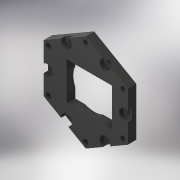
# Autodesk Inventor part: TA01
Saved by Autodesk Inventor 2017 (Build 210142000, 142)
## iProperties
Created: 2018-10-09
Part Number: TA01
Material: ABS Plastic
Document SubType Name: Modeling
Designer: Zach
Density: 1.06 g/cm^3
Appearance: Smooth - Black
Author: Zach
Autodesk Inventor part; units mm, degrees
ref_plane "YZ Plane" through (0, 0, 0) normal (1, 0, 0) x (0, 1, 0)
ref_plane "XZ Plane" through (0, 0, 0) normal (0, 1, 0) x (-1, 0, 0)
ref_plane "XY Plane" through (0, 0, 0) normal (0, 0, 1) x (1, 0, 0)
sketch "Sketch1" plane through (0, 0, 0) normal (0, 0, 1) x (1, 0, 0)
  circle A0 centre (0, 0) radius 12.5
  circle A1 centre (-30, 0) radius 3
  circle A2 centre (-15, -25.9808) radius 3
  circle A3 centre (15, -25.9808) radius 3
  circle A4 centre (30, 0) radius 3
  circle A5 centre (15, 25.9808) radius 3
  circle A6 centre (-15, 25.9808) radius 3
  line L0 (0, 57.5) -> (49.7965, 28.75)
  line L1 (49.7965, 28.75) -> (49.7965, -28.75)
  line L2 (49.7965, -28.75) -> (0, -57.5)
  line L3 (0, -57.5) -> (-49.7965, -28.75)
  line L4 (-49.7965, -28.75) -> (-49.7965, 28.75)
  line L5 (-49.7965, 28.75) -> (0, 57.5)
  point P0 (49.7965, 0)
  dimension "d0" = 25
  dimension "d2" = 6
  dimension "d6" = 360
  dimension "d15" = 30
  dimension "d33" = 115
  constraints: 12 end point, 7 centre point, 2 coincident, 2 horizontal alignment, 1 midpoint, 26 other
  measures "d0" diameter of A0
  measures "d2" diameter of A1
  measures "d15" distance of point (0, 0) A1.centre
  measures "d33" distance of L2.end L0.start
extrude "Extrusion1" add sketch "Sketch1" along normal blind 10 contours A1 | A2 | A3 | A4 | A5 | A6 | L0 L1 L2 L3 L4 L5
sketch "Sketch7" plane through (0, 0, 10) normal (0, 0, 1) x (1, 0, 0)
  circle A0 centre (0, 51) radius 3
  circle A1 centre (-44.1673, 25.5) radius 3
  circle A2 centre (-44.1673, -25.5) radius 3
  circle A3 centre (0, -51) radius 3
  circle A4 centre (44.1673, -25.5) radius 3
  circle A5 centre (44.1673, 25.5) radius 3
  line L0 (0, 51) -> (0, -51)
  point P0 (0, 0)
  dimension "d42" = 6
  dimension "d46" = 360
  dimension "d96" = 102
  constraints: 6 centre point, 2 end point, 1 vertical, 13 other
  measures "d42" diameter of A0
  measures "d96" distance of L0.start L0.end
extrude "Extrusion6" cut sketch "Sketch7" against normal through all
sketch "Sketch9" plane through (0, 0, 0) normal (0, 0, -1) x (-1, 0, 0)
  circle A0 centre (0, 0) radius 25
  dimension "d56" = 50
  constraints: 1 centre point, 1 coincident
  measures "d56" diameter of A0
extrude "Extrusion8" cut sketch "Sketch9" against normal blind 5
sketch "Sketch14" plane through (0, 0, 10) normal (0, 0, 1) x (1, 0, 0)
  circle A0 centre (-45.7965, 0) radius 2.5
  circle A1 centre (-22.8982, -39.6609) radius 2.5
  circle A2 centre (22.8982, -39.6609) radius 2.5
  circle A3 centre (45.7965, 0) radius 2.5
  circle A4 centre (22.8982, 39.6609) radius 2.5
  circle A5 centre (-22.8982, 39.6609) radius 2.5
  line L0 (-49.7965, 28.75) -> (-49.7965, -28.75) projected
  point P0 (0, 0)
  point P1 (-45.7965, 0)
  dimension "d81" = 5
  dimension "d85" = 360
  dimension "d97" = 4
  constraints: 6 centre point, 1 coincident, 1 horizontal alignment, 13 other
  measures "d81" diameter of A0
  measures "d97" distance from line of L0 A0.centre
extrude "Extrusion13" cut sketch "Sketch14" against normal through all
sketch "Sketch15" plane through (0, 0, 10) normal (0, 0, 1) x (1, 0, 0)
  circle A0 centre (-22.8982, 39.6609) radius 2.5 projected
  circle A1 centre (-22.8982, 39.6609) radius 6.5
  circle A2 centre (-45.7965, 0) radius 6.5
  circle A3 centre (-22.8982, -39.6609) radius 6.5
  circle A4 centre (22.8982, -39.6609) radius 6.5
  circle A5 centre (45.7965, 0) radius 6.5
  circle A6 centre (22.8982, 39.6609) radius 6.5
  point P0 (0, 0)
  dimension "d89" = 13
  dimension "d92" = 360
  constraints: 6 centre point, 1 coincident, 13 other
  measures "d89" diameter of A1
extrude "Extrusion14" cut sketch "Sketch15" against normal blind 5 contours A0 | A1 | A2 | A3 | A4 | A5 | A6
sketch "Sketch16" plane through (0, 0, 10) normal (0, 0, 1) x (1, 0, 0)
  line L0 (-22.6984, 22.6984) -> (31.2103, 22.6984)
  line L1 (31.2103, 22.6984) -> (31.2103, -22.6984)
  line L2 (31.2103, -22.6984) -> (-22.6984, -22.6984)
  line L3 (-22.6984, -22.6984) -> (-22.6984, 22.6984)
  point P0 (0, 0)
  constraints: 8 end point, 2 parallel, 1 horizontal, 1 perpendicular
extrude "Extrusion15" cut sketch "Sketch16" against normal through all
body "Solid1"
